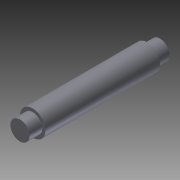
# Autodesk Inventor part: lower box weel shaft steel
Saved by Autodesk Inventor 2012 (Build 160160000, 160)
## iProperties
Created: 2012-12-28
Part Number: lower box weel shaft steel
Material: Default
Document SubType Name: Modeling
Designer: Bryce
Density: 1 g/cm^3
Author: Bryce
Autodesk Inventor part; units mm, degrees
ref_plane "YZ Plane" through (0, 0, 0) normal (1, 0, 0) x (0, 1, 0)
ref_plane "XZ Plane" through (0, 0, 0) normal (0, 1, 0) x (-1, 0, 0)
ref_plane "XY Plane" through (0, 0, 0) normal (0, 0, 1) x (1, 0, 0)
sketch "Sketch1" plane through (0, 0, 0) normal (0, 0, 1) x (1, 0, 0)
  circle A0 centre (0, 0) radius 6.35
  dimension "d0" = 12.7
  constraints: 1 centre point, 1 coincident
  measures "d0" diameter of A0
extrude "Extrusion1" add sketch "Sketch1" against normal blind 82.55
ref_plane "Work Plane4" through (0, 0, -12.7) normal (0, 0, 1) x (1, 0, 0)
sketch "Sketch4" plane through (0, 0, -12.7) normal (0, 0, 1) x (1, 0, 0)
  circle A0 centre (0, 0) radius 6.35 projected
  circle A1 centre (0, 0) radius 4.7625
  dimension "d27" = 9.525
  constraints: 1 centre point, 1 coincident
  measures "d27" diameter of A1
ref_plane "Work Plane5" through (0, 0, -69.85) normal (0, 0, -1) x (-1, 0, 0)
sketch "Sketch5" plane through (0, 0, -69.85) normal (0, 0, -1) x (-1, 0, 0)
  circle A0 centre (0, 0) radius 6.35 projected
  circle A1 centre (0, 0) radius 4.7625
  dimension "d24" = 9.525
  constraints: 1 centre point, 1 coincident
  measures "d24" diameter of A1
extrude "Extrusion6" cut sketch "Sketch5" along normal blind 25.4 contours A0 | A1
extrude "Extrusion7" cut sketch "Sketch4" along normal blind 25.4 contours A0 | A1
extrude "Extrusion8" add sketch "Sketch4" along normal blind 6.35 contours A1
extrude "Extrusion9" add sketch "Sketch5" along normal blind 6.35 contours A1
body "Solid1"
